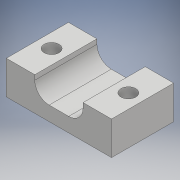
# Autodesk Inventor part: Uchwyt_na_silnik
Saved by Autodesk Inventor 2018 (Build 220112000, 112)
## iProperties
Created: 2019-08-02
Part Number: Uchwyt_na_silnik
Material: Ogólny
Document SubType Name: Modeling
Designer: Raven
Density: 1 g/cm^3
Appearance: Domyślna
Author: Raven
Autodesk Inventor part; units mm, degrees
ref_plane "YZ Plane" through (0, 0, 0) normal (1, 0, 0) x (0, 1, 0)
ref_plane "XZ Plane" through (0, 0, 0) normal (0, 1, 0) x (-1, 0, 0)
ref_plane "XY Plane" through (0, 0, 0) normal (0, 0, 1) x (1, 0, 0)
sketch "Szkic1" plane through (0, 0, 0) normal (0, 0, 1) x (1, 0, 0)
  line L0 (0, 0) -> (22, 0)
  line L1 (22, 0) -> (22, 13)
  line L2 (22, 13) -> (0, 13)
  line L3 (0, 13) -> (0, 0)
  dimension "d0" = 13
  dimension "d1" = 22
  constraints: 8 end point, 2 parallel, 1 horizontal, 1 perpendicular
  measures "d0" distance of L0.end L1.end
  measures "d1" distance of L1.end L2.end
extrude "Wyciągnięcie proste1" add sketch "Szkic1" along normal blind 7
sketch "Szkic2" plane through (0, 0, 7) normal (0, 0, 1) x (1, 0, 0)
  line L0 (22, 0) -> (22, 13) construction
  line L1 (0, 13) -> (0, 0) construction
  line L2 (22, 0) -> (16.05, 0) construction
  line L3 (16.05, 0) -> (16.05, 13) construction
  line L4 (16.05, 13) -> (22, 13) construction
  line L5 (22, 13) -> (22, 0) construction
  line L6 (0, 0) -> (22, 0) construction
  line L7 (0, 0) -> (5.95, 0) construction
  line L8 (5.95, 0) -> (5.95, 13) construction
  line L9 (5.95, 13) -> (0, 13) construction
  line L10 (0, 13) -> (0, 0) construction
  line L11 (16.05, 0) -> (5.95, 0)
  line L12 (5.95, 0) -> (5.95, 13)
  line L13 (5.95, 13) -> (16.05, 13)
  line L14 (16.05, 13) -> (16.05, 0)
  dimension "d4" = 5.95
  dimension "d5" = 5.95
  constraints: 24 end point, 6 parallel, 3 horizontal, 3 perpendicular, 1 point on line
  measures "d4" distance of L3.end L4.end
  measures "d5" distance of L9.end L8.end
extrude "Wyciągnięcie proste2" cut sketch "Szkic2" against normal blind 4
fillet "Zaokrąglenie1" radius 3 2 edges at (16.05, 6.5, 3) (5.95, 6.5, 3)
sketch "Szkic3" plane through (0, 0, 7) normal (0, 0, 1) x (1, 0, 0)
  line L0 (0, 0) -> (22, 0) construction
  line L1 (0, 0) -> (0, 6.5) construction
  line L2 (0, 13) -> (0, 0) construction
  line L3 (0, 6.5) -> (22, 6.5) construction
  line L4 (22, 0) -> (22, 13) construction
  line L5 (0, 6.5) -> (2.975, 6.5) construction
  line L6 (22, 6.5) -> (19.025, 6.5) construction
  circle A0 centre (2.975, 6.5) radius 1.55
  circle A1 centre (19.025, 6.5) radius 1.55
  dimension "d9" = 2.975
  dimension "d10" = 2.975
  dimension "d11" = 3.1
  dimension "d12" = 3.1
  constraints: 8 end point, 2 centre point, 2 coincident, 2 midpoint, 2 point on line
  measures "d9" distance of L1.end L5.end
  measures "d10" distance of L3.end L6.end
  measures "d11" diameter of A0
  measures "d12" diameter of A1
extrude "Wyciągnięcie proste3" cut sketch "Szkic3" against normal blind 7
equation "\"d12\" = d11"
